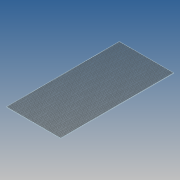
# Autodesk Inventor part: Boden2
Saved by Autodesk Inventor 2014 (Build 180170000, 170)
## iProperties
Created: 2013-02-25
Part Number: Boden2
Material: Stainless Steel
Document SubType Name: Modeling
Designer: Neef
Mass: 156.726 g
Surface Area: 490.24 cm^2
Volume: 19.3968 cm^3
Density: 8.08 g/cm^3
Appearance: Expanded Metal 01
Author: Neef
Autodesk Inventor part; units mm, degrees
ref_plane "YZ Plane" through (0, 0, 0) normal (1, 0, 0) x (0, 1, 0)
ref_plane "XZ Plane" through (0, 0, 0) normal (0, 1, 0) x (-1, 0, 0)
ref_plane "XY Plane" through (0, 0, 0) normal (0, 0, 1) x (1, 0, 0)
sketch "Skizze1" plane through (0, 0, 0) normal (0, 0, 1) x (1, 0, 0)
  line L0 (0, 105.232) -> (0, -209.068) projected
  line L1 (-65.2241, 0) -> (85.9759, 0) projected
  line L2 (-43.6241, 60.332) -> (64.3759, 60.332)
  line L3 (64.3759, 60.332) -> (64.3759, -164.168)
  line L4 (64.3759, -164.168) -> (-43.6241, -164.168)
  line L5 (-43.6241, -164.168) -> (-43.6241, 60.332)
  point P0 (0, 0)
  dimension "d0" = 108
  dimension "d1" = 224.5
  constraints: 8 end point, 2 parallel, 1 horizontal, 1 perpendicular
  measures "d0" distance of L2.start L2.end
  measures "d1" distance of L4.end L2.start
extrude "Extrusion1" add sketch "Skizze1" along normal blind 0.8
